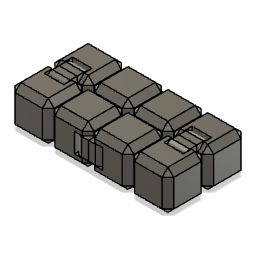
infinity_cube (Autodesk Fusion 360 design; units mm, degrees)
Autodesk Fusion 360 part; units mm, degrees
note: some values were not read from the file. Chosen so that the rebuilt part matches the saved one: which face or edge a step refers to.
sketch "BaseCubes" plane through (0, 0, 0) normal (0, 1, 0) x (1, 0, 0)
  line L0 (0, 0) -> (20, 0)
  line L1 (20, 0) -> (20, -20)
  line L2 (20, -20) -> (0, -20)
  line L3 (0, -20) -> (0, 0)
  line L4 (20.4, 0) -> (40.4, 0)
  line L5 (40.4, 0) -> (40.4, -20)
  line L6 (40.4, -20) -> (20.4, -20)
  line L7 (20.4, -20) -> (20.4, 0)
  dimension "d1" = 20
  dimension "d2" = 20
  dimension "d3" = 20
  dimension "d4" = 20
  dimension "d5" = 0.4
  constraint horizontal L0
  constraint vertical L1
  constraint horizontal L2
  constraint vertical L3
  constraint coincident L0.start L3.end
  constraint horizontal L4
  constraint vertical L5
  constraint horizontal L6
  constraint vertical L7
  constraint collinear L0 L4
  measures "d1" distance of L0.start L0.end
  measures "d2" distance of L0.start L2.end
  measures "d3" distance of L4.start L4.end
  measures "d4" distance of L4.start L6.end
  measures "d5" distance of L1 L7
extrude "Extrude1" add sketch "BaseCubes" along normal blind 20 contours L0 L1 L2 L3 makes body 1
extrude "Extrude2" add sketch "BaseCubes" along normal blind 20 separate body contours L4 L5 L6 L7 makes body 2
chamfer "Chamfer1" distance 3 angle 45 12 edges at (0, 0, 10) (20, 0, 10) (20, 10, 20) (10, 0, 20) (10, 0, 0) (20, 10, 0) (0, 20, 10) (10, 20, 20) (10, 20, 0) (20, 20, 10) (0, 10, 20) (0, 10, 0) 6 faces at (6.6667, 6.6667, 0) (0, 6.6667, 13.3333) (20, 6.6667, 6.6667) (6.6667, 20, 6.6667) (13.3333, 6.6667, 20) (6.6667, 0, 6.6667) on bodies 1
chamfer "Chamfer2" distance 3 angle 45 12 edges at (20.4, 20, 10) (30.4, 0, 0) (30.4, 20, 0) (20.4, 10, 20) (30.4, 20, 20) (40.4, 10, 20) (40.4, 0, 10) (40.4, 10, 0) (40.4, 20, 10) (20.4, 0, 10) (20.4, 10, 0) (30.4, 0, 20) 6 faces at (20.4, 6.6667, 13.3333) (27.0667, 20, 6.6667) (40.4, 6.6667, 6.6667) (27.0667, 6.6667, 0) (27.0667, 0, 6.6667) (33.7333, 6.6667, 20) on bodies 2
sketch "Hinge1" plane through (0, 20, 0) normal (0, 1, 0) x (-1, 0, 0)
  line L0 (-3, 17) -> (-17, 17)
  line L1 (-17, 17) -> (-17, 3)
  line L2 (-3, 3) -> (-3, 17)
  line L3 (-5, 0) -> (-15, 0)
  line L4 (-15, 0) -> (-15, 7)
  line L5 (-15, 7) -> (-5, 7)
  line L6 (-5, 7) -> (-5, 0)
  line L7 (-5.4, 6.6) -> (-14.6, 6.6)
  line L8 (-14.6, 6.6) -> (-14.6, -0.2)
  line L9 (-14.6, -0.2) -> (-5.4, -0.2)
  line L10 (-5.4, -0.2) -> (-5.4, 6.6)
  dimension "d12" = 10
  dimension "d13" = 7
  dimension "d14" = 10
  dimension "d15" = 2
  dimension "d16" = 9.2
  dimension "d17" = 6.8
  dimension "d18" = 0.4
  dimension "d19" = 0.4
  constraint horizontal L3
  constraint vertical L4
  constraint horizontal L5
  constraint vertical L6
  constraint horizontal L7
  constraint vertical L8
  constraint horizontal L9
  constraint vertical L10
  measures "d12" distance of L3.start L3.end
  measures "d13" distance of L3.start L5.end
  measures "d14" distance of L0 L5
  measures "d15" distance of L2 L6
  measures "d16" distance of L7.start L7.end
  measures "d17" distance of L7.start L9.end
  measures "d18" distance of L6 L10
  measures "d19" distance of L5 L7
sketch "Hinge2" plane through (0, 0, 20) normal (0, 0, 1) x (1, 0, 0)
  line L0 (37.4, 17) -> (23.4, 17)
  line L1 (23.4, 17) -> (23.4, 3)
  line L2 (23.4, 3) -> (37.4, 3)
  line L3 (33.4, 15) -> (40.4, 15)
  line L4 (40.4, 15) -> (40.4, 5)
  line L5 (40.4, 5) -> (33.4, 5)
  line L6 (33.4, 5) -> (33.4, 15)
  line L7 (33.8, 14.6) -> (40.6, 14.6)
  line L8 (40.6, 14.6) -> (40.6, 5.4)
  line L9 (40.6, 5.4) -> (33.8, 5.4)
  line L10 (33.8, 5.4) -> (33.8, 14.6)
  dimension "d20" = 7
  dimension "d21" = 10
  dimension "d22" = 10
  dimension "d23" = 2
  dimension "d24" = 6.8
  dimension "d25" = 9.2
  dimension "d26" = 0.4
  dimension "d27" = 0.4
  constraint horizontal L3
  constraint vertical L4
  constraint horizontal L5
  constraint vertical L6
  constraint horizontal L7
  constraint vertical L8
  constraint horizontal L9
  constraint vertical L10
  measures "d20" distance of L3.start L3.end
  measures "d21" distance of L3.start L5.end
  measures "d22" distance of L1 L6
  measures "d23" distance of L0 L3
  measures "d24" distance of L7.start L7.end
  measures "d25" distance of L7.start L9.end
  measures "d26" distance of L6 L10
  measures "d27" distance of L3 L7
sketch "Hinge3" plane through (0, 0, 0) normal (0, -1, 0) x (1, 0, 0)
  line L0 (17, 17) -> (3, 17)
  line L1 (3, 17) -> (3, 3)
  line L2 (3, 3) -> (17, 3)
  line L3 (13, 15) -> (20, 15)
  line L4 (20, 15) -> (20, 5)
  line L5 (20, 5) -> (13, 5)
  line L6 (13, 5) -> (13, 15)
  line L7 (13.4, 14.6) -> (20.2, 14.6)
  line L8 (20.2, 14.6) -> (20.2, 5.4)
  line L9 (20.2, 5.4) -> (13.4, 5.4)
  line L10 (13.4, 5.4) -> (13.4, 14.6)
  dimension "d28" = 7
  dimension "d29" = 10
  dimension "d30" = 2
  dimension "d31" = 10
  dimension "d32" = 6.8
  dimension "d33" = 9.2
  dimension "d34" = 0.4
  dimension "d35" = 0.4
  constraint horizontal L3
  constraint vertical L4
  constraint horizontal L5
  constraint vertical L6
  constraint horizontal L7
  constraint vertical L8
  constraint horizontal L9
  constraint vertical L10
  measures "d28" distance of L3.start L3.end
  measures "d29" distance of L3.start L5.end
  measures "d30" distance of L0 L3
  measures "d31" distance of L1 L6
  measures "d32" distance of L7.start L7.end
  measures "d33" distance of L7.start L9.end
  measures "d34" distance of L3 L7
  measures "d35" distance of L6 L10
sketch "Hinge4" plane through (0, 0, 0) normal (0, -1, 0) x (1, 0, 0)
  line L0 (37.4, 3) -> (37.4, 17)
  line L1 (37.4, 17) -> (23.4, 17)
  line L2 (23.4, 3) -> (37.4, 3)
  line L3 (20.4, 15) -> (27.4, 15)
  line L4 (27.4, 15) -> (27.4, 5)
  line L5 (27.4, 5) -> (20.4, 5)
  line L6 (20.4, 5) -> (20.4, 15)
  line L7 (20.2, 14.6) -> (27, 14.6)
  line L8 (27, 14.6) -> (27, 5.4)
  line L9 (27, 5.4) -> (20.2, 5.4)
  line L10 (20.2, 5.4) -> (20.2, 14.6)
  dimension "d36" = 7
  dimension "d37" = 10
  dimension "d38" = 2
  dimension "d39" = 10
  dimension "d40" = 6.8
  dimension "d41" = 9.2
  dimension "d42" = 0.4
  dimension "d43" = 0.4
  constraint horizontal L3
  constraint vertical L4
  constraint horizontal L5
  constraint vertical L6
  constraint horizontal L7
  constraint vertical L8
  constraint horizontal L9
  constraint vertical L10
  measures "d36" distance of L3.start L3.end
  measures "d37" distance of L3.start L5.end
  measures "d38" distance of L1 L3
  measures "d39" distance of L0 L4
  measures "d40" distance of L7.start L7.end
  measures "d41" distance of L7.start L9.end
  measures "d42" distance of L3 L7
  measures "d43" distance of L4 L8
extrude "Extrude3" cut sketch "Hinge1" against normal blind 7 contours L3 L4 L5 L6 L7 L8 L10 | L3 L7 L8 L10 bodies 1
extrude "Extrude4" add sketch "Hinge1" against normal blind 6.6 separate body contours L3 L8 L9 L10 | L3 L7 L8 L10 makes body 3
extrude "Extrude5" cut sketch "Hinge2" against normal blind 7 contours L3 L4 L5 L6 L7 L9 L10 | L4 L7 L9 L10 bodies 2
extrude "Extrude6" add sketch "Hinge2" against normal blind 6.6 separate body contours L4 L7 L8 L9 | L4 L7 L9 L10 makes body 4
extrude "Extrude7" cut sketch "Hinge3" sketch "Hinge4" against normal blind 7 contours L3 L4 L5 L6 L7 L9 L10 | L4 L7 L9 L10 of sketch 2 contours L3 L4 L5 L6 L7 L8 L9 | L6 L7 L8 L9 bodies 1 2
extrude "Extrude8" add sketch "Hinge3" against normal blind 6.6 separate body contours L4 L7 L8 L9 | L4 L7 L9 L10 makes body 5
extrude "Extrude9" add sketch "Hinge4" against normal blind 6.6 separate body contours L6 L7 L8 L9 | L6 L7 L9 L10 makes body 6
fillet "Fillet1" radius 3.3 2 edges at (10, 20, 6.6) (10, 13.4, 6.6) on bodies 3
fillet "Fillet2" radius 3.3 2 edges at (33.8, 10, 13.4) (33.8, 10, 20) on bodies 4
fillet "Fillet3" radius 3.3 4 edges at (13.4, 6.6, 10) (13.4, 0, 10) (27, 6.6, 10) (27, 0, 10) on bodies 5 6
sketch "PinCube1" plane through (15, 0, 0) normal (-1, 0, 0) x (0, 0, 1)
  line L0 (3, 20) -> (0, 17)
  line L1 (0, 17) -> (0, 13)
  line L2 (0, 13) -> (7, 13)
  line L3 (7, 13) -> (7, 20)
  line L4 (7, 20) -> (3, 20)
  circle A0 centre (3.5, 16.5) radius 1.3
  circle A1 centre (3.5, 16.5) radius 1.5
  dimension "d64" = 2.6
  dimension "d65" = 3
  dimension "d66" = 3.5
  dimension "d67" = 3.5
  constraint concentric A0 A1
  measures "d64" diameter of A0
  measures "d65" diameter of A1
  measures "d66" distance of L4 A0.centre
  measures "d67" distance of L1 A0.centre
sketch "PinHinge1" plane through (5.4, 0, 0) normal (-1, 0, 0) x (0, 0, 1)
  arc A0 (3.3, 13.4) -> (3.3, 20) centre (3.3, 16.7) ccw
  line L0 (3.3, 20) -> (-0.2, 20)
  line L1 (-0.2, 20) -> (-0.2, 13.4)
  line L2 (-0.2, 13.4) -> (3.3, 13.4)
  circle A1 centre (3.5, 16.5) radius 1.3
  circle A2 centre (3.5, 16.5) radius 1.5
  point P0 (3.5, 16.5)
  dimension "d68" = 2.6
  dimension "d69" = 3
  constraint coincident P0 A1.centre
  constraint concentric A1 A2
  measures "d68" diameter of A1
  measures "d69" diameter of A2
sketch "PinCube2" plane through (0, 5, 0) normal (0, 1, 0) x (-1, 0, 0)
  line L0 (-37.4, 20) -> (-40.4, 17)
  line L1 (-40.4, 17) -> (-40.4, 13)
  line L2 (-40.4, 13) -> (-33.4, 13)
  line L3 (-33.4, 13) -> (-33.4, 20)
  line L4 (-33.4, 20) -> (-37.4, 20)
  circle A0 centre (-36.9, 16.5) radius 1.3
  circle A1 centre (-36.9, 16.5) radius 1.5
  dimension "d70" = 2.6
  dimension "d71" = 3
  dimension "d72" = 3.5
  dimension "d73" = 3.5
  constraint concentric A0 A1
  measures "d70" diameter of A0
  measures "d71" diameter of A1
  measures "d72" distance of L1 A0.centre
  measures "d73" distance of L4 A0.centre
sketch "PinHinge2" plane through (0, 14.6, 0) normal (0, 1, 0) x (-1, 0, 0)
  arc A0 (-37.1, 13.4) -> (-37.1, 20) centre (-37.1, 16.7) ccw
  line L0 (-37.1, 20) -> (-40.6, 20)
  line L1 (-40.6, 20) -> (-40.6, 13.4)
  line L2 (-40.6, 13.4) -> (-37.1, 13.4)
  circle A1 centre (-36.9, 16.5) radius 1.5
  circle A2 centre (-36.9, 16.5) radius 1.3
  point P0 (-36.9, 16.5)
  dimension "d74" = 3
  dimension "d75" = 2.6
  constraint coincident P0 A1.centre
  constraint concentric A1 A2
  measures "d74" diameter of A1
  measures "d75" diameter of A2
sketch "PinCube3" plane through (0, 0, 5) normal (0, 0, 1) x (1, 0, 0)
  line L0 (17, 0) -> (20, 3)
  line L1 (20, 3) -> (20, 7)
  line L2 (20, 7) -> (13, 7)
  line L3 (13, 7) -> (13, 0)
  line L4 (13, 0) -> (17, 0)
  circle A0 centre (16.5, 3.5) radius 1.3
  circle A1 centre (16.5, 3.5) radius 1.5
  dimension "d76" = 2.6
  dimension "d77" = 3
  dimension "d78" = 3.5
  dimension "d79" = 3.5
  constraint concentric A0 A1
  measures "d76" diameter of A0
  measures "d77" diameter of A1
  measures "d78" distance of L1 A0.centre
  measures "d79" distance of L4 A0.centre
sketch "PinHinge3" plane through (0, 0, 14.6) normal (0, 0, 1) x (1, 0, 0)
  arc A0 (16.7, 6.6) -> (16.7, 0) centre (16.7, 3.3) ccw
  line L0 (16.7, 0) -> (20.2, 0)
  line L1 (20.2, 0) -> (20.2, 6.6)
  line L2 (20.2, 6.6) -> (16.7, 6.6)
  circle A1 centre (16.5, 3.5) radius 1.3
  circle A2 centre (16.5, 3.5) radius 1.5
  point P0 (16.5, 3.5)
  dimension "d80" = 2.6
  dimension "d81" = 3
  constraint coincident P0 A1.centre
  measures "d80" diameter of A1
  measures "d81" diameter of A2
sketch "PinCube4" plane through (0, 0, 15) normal (0, 0, -1) x (-1, 0, 0)
  line L0 (-23.4, 0) -> (-20.4, 3)
  line L1 (-20.4, 3) -> (-20.4, 7)
  line L2 (-20.4, 7) -> (-27.4, 7)
  line L3 (-27.4, 7) -> (-27.4, 0)
  line L4 (-27.4, 0) -> (-23.4, 0)
  circle A0 centre (-23.9, 3.5) radius 1.3
  circle A1 centre (-23.9, 3.5) radius 1.5
  dimension "d82" = 2.6
  dimension "d83" = 3
  dimension "d84" = 3.5
  dimension "d85" = 3.5
  constraint concentric A0 A1
  measures "d82" diameter of A0
  measures "d83" diameter of A1
  measures "d84" distance of L4 A0.centre
  measures "d85" distance of L1 A0.centre
sketch "PinHinge4" plane through (0, 0, 5.4) normal (0, 0, -1) x (-1, 0, 0)
  arc A0 (-23.7, 6.6) -> (-23.7, 0) centre (-23.7, 3.3) ccw
  line L0 (-23.7, 0) -> (-20.2, 0)
  line L1 (-20.2, 0) -> (-20.2, 6.6)
  line L2 (-20.2, 6.6) -> (-23.7, 6.6)
  circle A1 centre (-23.9, 3.5) radius 1.3
  circle A2 centre (-23.9, 3.5) radius 1.5
  point P0 (-23.9, 3.5)
  dimension "d86" = 2.6
  dimension "d87" = 3
  constraint coincident P0 A1.centre
  measures "d86" diameter of A1
  measures "d87" diameter of A2
extrude "Extrude10" cut sketch "PinCube1" along normal blind 3 draft -25 contours A0 | A1 bodies 3
extrude "Extrude11" add sketch "PinCube1" along normal blind 3 draft -30 contours A0 bodies 1
extrude "Extrude12" cut sketch "PinHinge1" along normal blind 3 draft -25 contours A1 | A2 bodies 1
extrude "Extrude13" add sketch "PinHinge1" along normal blind 3 draft -30 contours A1 bodies 3
extrude "Extrude14" cut sketch "PinHinge2" along normal blind 3 draft -25 contours A1 | A2 bodies 2
extrude "Extrude15" add sketch "PinHinge2" along normal blind 3 draft -30 contours A2 bodies 4
extrude "Extrude16" cut sketch "PinCube2" along normal blind 3 draft -25 contours A0 | A1 bodies 4
extrude "Extrude17" add sketch "PinCube2" along normal blind 3 draft -30 contours A0 bodies 2
extrude "Extrude18" cut sketch "PinCube4" along normal blind 3 draft -25 contours A0 | A1 bodies 6
extrude "Extrude19" add sketch "PinCube4" along normal blind 3 draft -30 contours A0 bodies 2
extrude "Extrude20" cut sketch "PinHinge4" along normal blind 3 draft -25 contours A1 | A2 bodies 2
extrude "Extrude21" add sketch "PinHinge4" along normal blind 3 draft -30 contours A1 bodies 6
extrude "Extrude22" cut sketch "PinCube3" along normal blind 3 draft -25 contours A0 | A1 bodies 5
extrude "Extrude23" add sketch "PinCube3" along normal blind 3 draft -30 contours A0 bodies 1
extrude "Extrude24" cut sketch "PinHinge3" along normal blind 3 draft -25 contours A1 | A2 bodies 1
extrude "Extrude25" add sketch "PinHinge3" along normal blind 3 draft -30 contours A1 bodies 5
mirror "Mirror1" about plane through (14.6, 20, -0.2) normal (0, 0, -1) of bodies 1 3 5 makes body 7 at (0, 7.6667, -12.7333) makes body 8 at (11.5333, 17.8, -0.2) makes body 9 at (20.2, 4.4, -11.9333)
mirror "Mirror2" about plane through (40.6, 14.6, 20) normal (1, 0, 0) of bodies 2 4 6 makes body 10 at (53.1333, 7.6667, 0) makes body 11 at (40.6, 11.5333, 17.8) makes body 12 at (61, 2.2, 8.4667)
ref_plane "WorkPlane1" through (30.4, 10, -0.2) normal (0, 0, -1) x (-1, 0, 0)
mirror "Mirror3" about plane through (30.4, 10, -0.2) normal (0, 0, -1) of bodies 2 4 6 10 11 12 makes body 13 at (28.0667, 7.6667, -0.4) makes body 14 at (36.9424, 8.4667, -13.8037) makes body 15 at (20.2, 2.2, -8.8667) makes body 16 at (53.1333, 7.6667, -0.4) makes body 17 at (44.2576, 8.4667, -13.8037) makes body 18 at (61, 2.2, -8.8667)
copy_body "CopyPasteBodies1" bodies 1 3 5 7 8 9 makes body 19 makes body 20 makes body 21 makes body 22 makes body 23 makes body 24
move_body "Move1" bodies 19 20 21 22 23 24 to x (-1, 0, 0) y (0, 1, 0) z (0, 0, -1) at (0, 0, 0)
move_body "Move2" bodies 19 20 21 22 23 24 to x (1, 0, 0) y (0, 1, 0) z (0, 0, 1) at (81.2, 0, -0.4)
